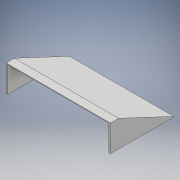
# Autodesk Inventor part: Front_Chassi
Saved by Autodesk Inventor 2018.2 (Build 222227000, 227)
## iProperties
Created: 2018-08-12
Part Number: Front_Chassi
Material: Generic
Document SubType Name: Modeling
Designer: mateu
Density: 1 g/cm^3
Appearance: Default
Author: mateu
Autodesk Inventor part; units mm, degrees
ref_plane "YZ Plane" through (0, 0, 0) normal (1, 0, 0) x (0, 1, 0)
ref_plane "XZ Plane" through (0, 0, 0) normal (0, 1, 0) x (-1, 0, 0)
ref_plane "XY Plane" through (0, 0, 0) normal (0, 0, 1) x (1, 0, 0)
sketch "Sketch1" plane through (0, 0, 0) normal (0, 0, 1) x (1, 0, 0)
  line L0 (0, 0) -> (0, 85)
  line L1 (0, 85) -> (160, 85)
  line L2 (160, 85) -> (160, 0)
  line L3 (160, 0) -> (157.6, 0)
  line L4 (157.6, 0) -> (157.6, 82.6)
  line L5 (157.6, 82.6) -> (2.4, 82.6)
  line L6 (2.4, 82.6) -> (2.4, 0)
  line L7 (2.4, 0) -> (0, 0)
  dimension "d0" = 85
  dimension "d1" = 160
  dimension "d2" = 2.4
  dimension "d3" = 82.6
  dimension "d4" = 155.2
  constraints: 16 end point, 6 perpendicular, 1 parallel, 1 point on line, 1 vertical
  measures "d0" distance of L0.start L0.end
  measures "d1" distance of L0.end L1.end
  measures "d2" distance of L2.end L3.end
  measures "d3" distance of L3.end L4.end
  measures "d4" distance of L4.end L5.end
extrude "Extrusion1" add sketch "Sketch1" along normal blind 0.9
sketch "Sketch2" plane through (0, 0, 0) normal (-1, 0, 0) x (0, 0, 1)
  line L0 (0, 0) -> (0.9, 0) projected
  line L1 (0.9, 0) -> (40.9, 0)
  line L2 (0.9, 0) -> (0.9, 85) projected
  line L3 (0.9, 85) -> (0.9, 0)
  line L4 (40.9, 0) -> (110.9, 0) construction
  line L5 (0.9, 85) -> (0.9, 0) projected
  line L6 (40.9, 0) -> (0.9, 85)
  dimension "d7" = 40
  constraints: 8 end point, 2 horizontal, 1 perpendicular
  measures "d7" distance of L0.end L1.end
extrude "Extrusion2" add sketch "Sketch2" against normal blind 2.4
sketch "Sketch3" plane through (160, 0, 0) normal (1, 0, 0) x (0, 0, -1)
  line L0 (-0.9, 0) -> (-0.9, 85) projected
  line L1 (-0.9, 0) -> (-30.8653, 0)
  line L2 (0, 0) -> (-40.9, 0) projected
  line L3 (-0.9, 0) -> (-40.9, 0)
  line L4 (0, 85) -> (-0.9, 85) projected
  line L5 (-0.9, 85) -> (-0.9, 0)
  line L6 (0, 0) -> (-40.9, 0) projected
  line L7 (-0.9, 85) -> (-40.9, 0) projected
  line L8 (-0.9, 85) -> (-40.9, 0)
  constraints: 8 end point, 2 collinear, 1 horizontal, 1 perpendicular
extrude "Extrusion3" add sketch "Sketch3" against normal blind 2.4
sketch "Sketch5" plane through (2.4, 0, 0) normal (1, 0, 0) x (0, 0, -1)
  line L0 (0, 0) -> (-40.9, 0) projected
  line L1 (-40.9, 0) -> (-0.9, 85)
  line L2 (-0.9, 85) -> (-0.9, 82.6) projected
  line L3 (-0.9, 85) -> (-0.9, 82.6)
  line L4 (-0.9, 82.6) -> (-39.7706, 0)
  line L5 (-39.7706, 0) -> (-40.9, 0)
  constraints: 8 end point, 2 collinear, 1 parallel
extrude "Extrusion5" add sketch "Sketch5" along normal blind 156
sketch "Sketch6" plane through (0, 0, 40.9) normal (0, -1, 0) x (1, 0, 0)
  line L0 (0, -40.9) -> (160, -40.9) projected
  line L1 (0, 0) -> (0, -40) projected
  line L2 (0, -40.9) -> (0, 0)
  line L3 (0, 0) -> (160, 0) projected
  line L4 (0, 0) -> (160, 0)
  line L5 (160, -40.9) -> (160, 0) projected
  line L6 (160, 0) -> (160, -40.9)
  line L7 (157.6, -40.9) -> (157.6, -1.1294) projected
  line L8 (160, -40.9) -> (157.6, -40.9)
  line L9 (157.6, -40.9) -> (157.6, -1.1294)
  line L10 (2.4, -1.1294) -> (157.6, -1.1294) projected
  line L11 (157.6, -1.1294) -> (2.4, -1.1294)
  line L12 (2.4, -1.1294) -> (2.4, -40.9)
  line L13 (2.4, -40.9) -> (0, -40.9)
  constraints: 16 end point, 6 perpendicular, 2 collinear, 1 point on line
extrude "Extrusion6" add sketch "Sketch6" along normal blind 12.6 contours L2 L1 L3 L5 L0 L7 L10 L12
body "Solid1"
